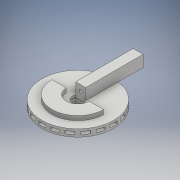
# Autodesk Inventor part: Parcial3_Repo
Saved by Autodesk Inventor 2018 (Build 220112000, 112)
## iProperties
Created: 2020-06-28
Part Number: Parcial3_Repo
Material: Generic
Document SubType Name: Modeling
Designer: Ivan
Density: 1 g/cm^3
Appearance: Default
Author: Ivan
Autodesk Inventor part; units mm, degrees
ref_plane "YZ Plane" through (0, 0, 0) normal (1, 0, 0) x (0, 1, 0)
ref_plane "XY Plane" through (0, 0, 0) normal (0, 0, 1) x (1, 0, 0)
sketch "Sketch1" plane through (0, 0, 0) normal (0, 0, 1) x (1, 0, 0)
  circle A0 centre (0, 0) radius 25
  circle A1 centre (0, 0) radius 4
  line L0 (-3.4641, 2) -> (3.4641, 2)
  dimension "d0" = 50
  dimension "d1" = 8
  dimension "d2" = 2
  constraints: 2 centre point, 2 coincident, 2 end point, 2 point on circle, 1 horizontal
  measures "d0" diameter of A0
  measures "d1" diameter of A1
  measures "d2" distance centre to line of A1 L0
extrude "Extrusion1" add sketch "Sketch1" along normal blind 5 contours A0 | L0 A1 picked at (-0.1548, 2.6577)
ref_plane "Work Plane1" through (0, 25, 0) normal (0, 1, 0) x (-1, 0, 0)
sketch "Sketch3" plane through (0, 25, 0) normal (0, 1, 0) x (-1, 0, 0)
  line L0 (2.5, 1.5) -> (-2.5, 1.5)
  line L1 (-2.5, 1.5) -> (-2.5, 3.5)
  line L2 (-2.5, 3.5) -> (2.5, 3.5)
  line L3 (2.5, 3.5) -> (2.5, 1.5)
  line L4 (25, 0) -> (25, 5) construction
  point P0 (0, 0)
  point P1 (0, 1.5)
  point P2 (2.5, 2.5)
  point P3 (25, 2.5)
  dimension "d12" = 5
  dimension "d13" = 2
  constraints: 8 end point, 3 midpoint, 2 parallel, 1 horizontal, 1 horizontal alignment, 1 perpendicular, 1 vertical alignment
  measures "d12" distance of L0.start L0.end
  measures "d13" distance of L0.end L1.end
extrude "Extrusion2" cut sketch "Sketch3" against normal blind 25
pattern_circular "Circular Pattern1" count 20 over 360 about axis through (0, 0, -10) along (0, 0, 1) of "Extrusion2"
sketch "Sketch4" plane through (0, 0, 5) normal (0, 0, 1) x (1, 0, 0)
  line L0 (-3.4641, 2) -> (3.4641, 2) projected
  line L1 (-3.4641, 2) -> (3.4641, 2)
  line L2 (3.4641, 2) -> (3.4641, 42)
  line L3 (3.4641, 42) -> (-3.4641, 42)
  line L4 (-3.4641, 42) -> (-3.4641, 2)
  point P0 (0, 0)
  dimension "d19" = 40
  dimension "d20" = 6.9282
  constraints: 8 end point, 2 parallel, 1 horizontal, 1 perpendicular
  measures "d19" distance between parallel lines of L0 L3
  measures "d20" distance between parallel lines of L4 L2
extrude "Extrusion3" add sketch "Sketch4" along normal blind 8
sketch "Sketch5" plane through (-3.4641, 42, 5) normal (0, 1, 0) x (1, 0, 0)
  circle A0 centre (3.4641, -4) radius 2
  line L0 (6.9282, 0) -> (0, 0) construction
  line L1 (0, 0) -> (0, -8) construction
  line L2 (6.9282, -8) -> (0, -8) construction
  line L3 (6.9282, 0) -> (6.9282, -8) construction
  point P0 (3.4641, 5)
  point P1 (6.9282, -4)
  point P2 (3.4641, -8)
  dimension "d23" = 4
  constraints: 2 midpoint, 1 centre point, 1 horizontal alignment, 1 vertical alignment
  measures "d23" diameter of A0
sketch "Sketch6" plane through (-3.4641, 2, 3.5) normal (0, -1, 0) x (1, 0, 0)
  circle A0 centre (3.4641, 5.5) radius 1
  line L0 (0, 9.5) -> (6.9282, 9.5) projected
  line L1 (6.9282, 1.5) -> (6.9282, 9.5) projected
  point P0 (3.4641, -3.5)
  point P1 (3.4641, 9.5)
  point P2 (6.9282, 5.5)
  dimension "d24" = 2
  constraints: 2 midpoint, 1 centre point, 1 horizontal alignment, 1 vertical alignment
  measures "d24" diameter of A0
loft "Loft1" cut profiles "Sketch5", "Sketch6"
sketch "Sketch7" plane through (0, 0, 0) normal (0, 1, 0) x (-1, 0, 0)
  line L0 (25, 5) -> (-25, 5) construction
  line L1 (8, 5) -> (18, 5)
  line L2 (18, 5) -> (18, 8)
  line L3 (18, 8) -> (8, 8)
  line L4 (8, 8) -> (8, 5)
  line L5 (-10.0643, 3.5) -> (-5.3091, 3.5) construction
  line L6 (-5.3091, 3.5) -> (-5.3091, 1.5) construction
  line L7 (-5.3091, 1.5) -> (-10.0643, 1.5) construction
  line L8 (-10.0643, 1.5) -> (-10.0643, 3.5) construction
  line L9 (-24.8747, 1.5) -> (-24.8747, 1.5) construction
  line L10 (-24.8747, 1.5) -> (-24.8747, 3.5) construction
  line L11 (-24.8747, 3.5) -> (-24.8747, 3.5) construction
  line L12 (-24.8747, 3.5) -> (-24.8747, 1.5) construction
  line L13 (-24.4298, 1.5) -> (-22.8847, 1.5) construction
  line L14 (-22.8847, 1.5) -> (-22.8847, 3.5) construction
  line L15 (-22.8847, 3.5) -> (-24.4298, 3.5) construction
  line L16 (-24.4298, 3.5) -> (-24.4298, 1.5) construction
  line L17 (-21.5935, 1.5) -> (-18.6546, 1.5) construction
  line L18 (-18.6546, 1.5) -> (-18.6546, 3.5) construction
  line L19 (-18.6546, 3.5) -> (-21.5935, 3.5) construction
  line L20 (-21.5935, 3.5) -> (-21.5935, 1.5) construction
  line L21 (-16.6435, 1.5) -> (-12.5984, 1.5) construction
  line L22 (-12.5984, 1.5) -> (-12.5984, 3.5) construction
  line L23 (-12.5984, 3.5) -> (-16.6435, 3.5) construction
  line L24 (-16.6435, 3.5) -> (-16.6435, 1.5) construction
  line L25 (-10.0643, 1.5) -> (-5.3091, 1.5) construction
  line L26 (-5.3091, 1.5) -> (-5.3091, 3.5) construction
  line L27 (-5.3091, 3.5) -> (-10.0643, 3.5) construction
  line L28 (-10.0643, 3.5) -> (-10.0643, 1.5) construction
  line L29 (10.0643, 1.5) -> (5.3091, 1.5) construction
  line L30 (5.3091, 1.5) -> (5.3091, 3.5) construction
  line L31 (5.3091, 3.5) -> (10.0643, 3.5) construction
  line L32 (10.0643, 3.5) -> (10.0643, 1.5) construction
  line L33 (-12.5984, 1.5) -> (-16.6435, 1.5) construction
  line L34 (-16.6435, 1.5) -> (-16.6435, 3.5) construction
  line L35 (-16.6435, 3.5) -> (-12.5984, 3.5) construction
  line L36 (-12.5984, 3.5) -> (-12.5984, 1.5) construction
  line L37 (-18.6546, 1.5) -> (-21.5935, 1.5) construction
  line L38 (-21.5935, 1.5) -> (-21.5935, 3.5) construction
  line L39 (-21.5935, 3.5) -> (-18.6546, 3.5) construction
  line L40 (-18.6546, 3.5) -> (-18.6546, 1.5) construction
  line L41 (-22.8847, 1.5) -> (-24.4298, 1.5) construction
  line L42 (-24.4298, 1.5) -> (-24.4298, 3.5) construction
  line L43 (-24.4298, 3.5) -> (-22.8847, 3.5) construction
  line L44 (-22.8847, 3.5) -> (-22.8847, 1.5) construction
  line L45 (12.5984, 3.5) -> (16.6435, 3.5) construction
  line L46 (16.6435, 3.5) -> (16.6435, 1.5) construction
  line L47 (16.6435, 1.5) -> (12.5984, 1.5) construction
  line L48 (12.5984, 1.5) -> (12.5984, 3.5) construction
  line L49 (18.6546, 3.5) -> (21.5935, 3.5) construction
  line L50 (21.5935, 3.5) -> (21.5935, 1.5) construction
  line L51 (21.5935, 1.5) -> (18.6546, 1.5) construction
  line L52 (18.6546, 1.5) -> (18.6546, 3.5) construction
  line L53 (22.8847, 3.5) -> (24.4298, 3.5) construction
  line L54 (24.4298, 3.5) -> (24.4298, 1.5) construction
  line L55 (24.4298, 1.5) -> (22.8847, 1.5) construction
  line L56 (22.8847, 1.5) -> (22.8847, 3.5) construction
  line L57 (24.8747, 3.5) -> (24.8747, 3.5) construction
  line L58 (24.8747, 3.5) -> (24.8747, 1.5) construction
  line L59 (24.8747, 1.5) -> (24.8747, 1.5) construction
  line L60 (24.8747, 1.5) -> (24.8747, 3.5) construction
  line L61 (24.4298, 3.5) -> (22.8847, 3.5) construction
  line L62 (22.8847, 3.5) -> (22.8847, 1.5) construction
  line L63 (22.8847, 1.5) -> (24.4298, 1.5) construction
  line L64 (24.4298, 1.5) -> (24.4298, 3.5) construction
  line L65 (21.5935, 3.5) -> (18.6546, 3.5) construction
  line L66 (18.6546, 3.5) -> (18.6546, 1.5) construction
  line L67 (18.6546, 1.5) -> (21.5935, 1.5) construction
  line L68 (21.5935, 1.5) -> (21.5935, 3.5) construction
  line L69 (16.6435, 3.5) -> (12.5984, 3.5) construction
  line L70 (12.5984, 3.5) -> (12.5984, 1.5) construction
  line L71 (12.5984, 1.5) -> (16.6435, 1.5) construction
  line L72 (16.6435, 1.5) -> (16.6435, 3.5) construction
  line L73 (10.0643, 3.5) -> (5.3091, 3.5) construction
  line L74 (5.3091, 3.5) -> (5.3091, 1.5) construction
  line L75 (5.3091, 1.5) -> (10.0643, 1.5) construction
  line L76 (10.0643, 1.5) -> (10.0643, 3.5) construction
  line L77 (2.5, 3.5) -> (-2.5, 3.5) construction
  line L78 (-2.5, 3.5) -> (-2.5, 1.5) construction
  line L79 (-2.5, 1.5) -> (2.5, 1.5) construction
  line L80 (2.5, 1.5) -> (2.5, 3.5) construction
  line L81 (-2.5, 3.5) -> (2.5, 3.5) construction
  line L82 (2.5, 3.5) -> (2.5, 1.5) construction
  line L83 (2.5, 1.5) -> (-2.5, 1.5) construction
  line L84 (-2.5, 1.5) -> (-2.5, 3.5) construction
  line L85 (3.4641, 5) -> (-3.4641, 5) construction
  line L86 (-3.4641, 5) -> (3.4641, 5) construction
  line L87 (-25, 0) -> (25, 0) construction
  circle A0 centre (0, 9) radius 1 construction
  line L88 (3.4641, 3.5) -> (-3.4641, 3.5) construction
  line L89 (-3.4641, 3.5) -> (-3.4641, 5) construction
  line L90 (-3.4641, 5) -> (-3.4641, 13) construction
  line L91 (3.4641, 13) -> (-3.4641, 13) construction
  line L92 (3.4641, 5) -> (3.4641, 13) construction
  line L93 (3.4641, 3.5) -> (3.4641, 5) construction
  line L94 (0, -2.6) -> (0, 15.6) projected
  point P0 (0, 0)
  dimension "d29" = 8
  dimension "d30" = 3
  dimension "d31" = 10
  constraints: 8 end point, 2 parallel, 1 horizontal, 1 perpendicular, 1 point on line
  measures "d29" distance from line of A0.centre L4
  measures "d30" distance between parallel lines of L0 L3
  measures "d31" distance between parallel lines of L2 L4
revolve "Revolution1" add sketch "Sketch7" angle 180 about axis through (0, 0, -10) along (0, 0, 1)
body "Solid1"
